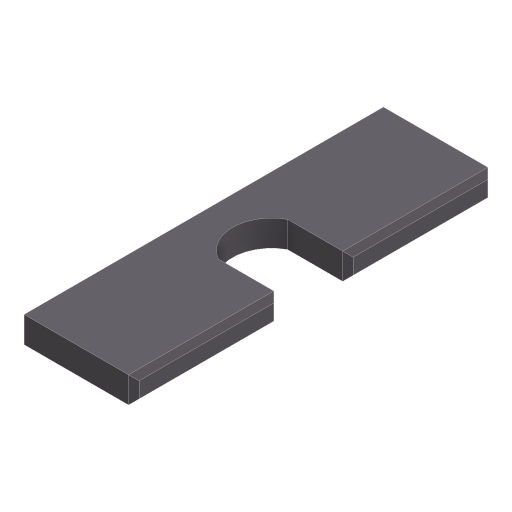
# Autodesk Inventor part: ProbeHead_Kabelfixieung_V1
Saved by Autodesk Inventor 2023.2 (Build 272271000, 271)
## iProperties
Created: 2024-06-19
Part Number: ProbeHead_Kabelfixieung_V1
Material: Generisch
Document SubType Name: Modeling
Designer: Nils Bade
Density: 1 g/cm^3
Appearance: ABS-Farbe
Author: Nils Bade
Autodesk Inventor part; units mm, degrees
ref_plane "YZ Plane" through (0, 0, 0) normal (1, 0, 0) x (0, 1, 0)
ref_plane "XZ Plane" through (0, 0, 0) normal (0, 1, 0) x (-1, 0, 0)
ref_plane "XY Plane" through (0, 0, 0) normal (0, 0, 1) x (1, 0, 0)
sketch "S-Base" plane through (0, 0, 0) normal (0, 1, 0) x (-1, 0, 0)
  line L0 (0, 0) -> (11, 0)
  line L1 (11, 0) -> (11, -34.4)
  line L2 (11, -34.4) -> (0, -34.4)
  line L3 (0, -34.4) -> (0, 0)
  circle A0 centre (4, -17.2) radius 3.5
  line L4 (0, -13.9) -> (7.5, -13.9)
  line L5 (7.5, -13.9) -> (7.5, -20.5)
  line L6 (7.5, -20.5) -> (0, -20.5)
  line L7 (0, -20.5) -> (0, -13.9) construction
  line L8 (7.5, -17.2) -> (0, -17.2) construction
  circle A1 centre (4, -17.2) radius 3.75
  point P0 (5.7812, -20.5)
  point P1 (5.7812, -13.9)
  dimension "d1" = 7
  dimension "d0" = 34.4
  dimension "d2" = 17.2
  dimension "d3" = 6.6
  dimension "d4" = 11
  dimension "d5" = 7.5
  dimension "d6" = 0.25
  constraints: 18 end point, 4 parallel, 2 horizontal, 2 midpoint, 2 perpendicular, 2 point on line, 1 centre point, 1 horizontal alignment, 2 other
  measures "d0" distance between parallel lines of L2 L0
  measures "d2" distance between parallel lines of L2 L8
  measures "d3" distance between parallel lines of L4 L6
  measures "d4" distance between parallel lines of L3 L1
  measures "d5" distance between parallel lines of L3 L5
extrude "Ex-Base" add sketch "S-Base" along normal blind 2.5 contours L0 L1 L2 L3 L6 A1 L5 L4 | A1 L4 A0 | L6 A0 A1 | A0 L4 | L4 L5 A1 | L6 A0 | A1 L5 L6
chamfer "Fase1" distance 0.5 angle 45 12 edges at (-11, 1.25, 0) (0, 1.25, 0) (0, 1.25, -34.4) (-11, 1.25, -34.4) (0, 1.25, -20.5) (0, 1.25, -13.9) (-11, 2.5, -17.2) (-11, 0, -17.2) (0, 2.5, -6.95) (0, 0, -6.95) (0, 2.5, -27.45) (0, 0, -27.45)
equation "\"d2\" = 0.5 * d0"
